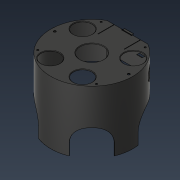
# Autodesk Inventor part: Gehäuse Mantel
Saved by Autodesk Inventor 2022.3 (Build 263350000, 350)
## iProperties
Part Number: Gehäuse Mantel
Material: Polyethylen, hohe Dichte
Document SubType Name: Modeling
Designer: rYan
Density: 0.952 g/cm^3
Appearance: Glatt - Schwarz
Mass: 76.0601 g
Surface Area: 1373.15 cm^2
Volume: 79.895 cm^3
Author: rYan
Autodesk Inventor part; units mm, degrees
ref_plane "XZ Plane" through (0, 0, 0) normal (0, 1, 0) x (-1, 0, 0)
ref_plane "XY Plane" through (0, 0, 0) normal (0, 0, 1) x (1, 0, 0)
sketch "Skizze1" plane through (0, 0, 0) normal (0, 0, 1) x (1, 0, 0)
  arc A0 (-44.0306, 77) -> (44.0306, 77) centre (0, 0) ccw
  circle A1 centre (0, 0) radius 25
  circle A2 centre (54.772, 35) radius 20
  circle A3 centre (-54.772, 35) radius 20
  circle A4 centre (-35, -54.772) radius 20
  circle A5 centre (35, -54.772) radius 20
  line L0 (0, 110.14) -> (0, -121.84) projected
  line L1 (-124.18, 0) -> (124.18, 0) projected
  line L2 (-44.0306, 77) -> (44.0306, 77)
  circle A6 centre (0, -59.5) radius 7.5
  circle A7 centre (0, 59.5) radius 7.5
  circle A8 centre (-80, 0) radius 2.2
  circle A9 centre (80, 0) radius 2.2
  dimension "d0" = 177.4
  dimension "d1" = 50
  dimension "d2" = 40
  dimension "d3" = 35
  dimension "d4" = 54.772
  dimension "d5" = 54.772
  dimension "d6" = 35
  dimension "d7" = 77
  dimension "d16" = 59.5
  dimension "d17" = 15
  dimension "d85" = 4.4
  dimension "d86" = 160
  constraints: 10 centre point, 4 point on line, 2 coincident, 2 end point, 2 equal radius, 2 point on circle, 1 horizontal, 4 other
  measures "d0" diameter of A0
  measures "d1" diameter of A1
  measures "d2" diameter of A2
  measures "d3" distance from line of A2.centre L1
  measures "d4" distance from line of A2.centre L0
  measures "d5" distance from line of L1 A5.centre
  measures "d6" distance from line of A5.centre L0
  measures "d7" distance between parallel lines of L2 L1
  measures "d16" distance from line of A6.centre L1
  measures "d17" diameter of A6
  measures "d85" diameter of A8
  measures "d86" distance of A9.centre A8.centre
extrude "Extrusion1" add sketch "Skizze1" along normal blind 1.2 contours L2 L0 A7 A1 L1 A8 A0 | L1 A8 A1 L0 A6 A0 | L2 A0 L1 A9 A1 L0 A7 | L0 A6 A1 L1 A9 A0 | A7 L0 | L0 A7 | A6 L0 | L0 A6
sketch "Skizze5" plane through (0, 0, 0) normal (0, 0, -1) x (-1, 0, 0)
  line L0 (-44.0306, 77) -> (44.0306, 77) projected
  line L1 (-29, 77) -> (29, 77)
  line L2 (29, 77) -> (29, -29)
  line L3 (-29, -29) -> (-29, 77)
  line L4 (0, -121.84) -> (0, 110.14) projected
  line L5 (-29, -29) -> (29, -29)
  circle A0 centre (0, 0) radius 25 projected
  circle A1 centre (-35, -54.772) radius 20 projected
  circle A2 centre (35, -54.772) radius 20 projected
  circle A3 centre (54.772, 35) radius 20 projected
  circle A4 centre (-54.772, 35) radius 20 projected
  arc A5 (-44.0306, 77) -> (44.0306, 77) centre (0, 0) ccw projected
  line L6 (-44.0306, 77) -> (44.0306, 77) projected
  circle A6 centre (-54.772, 35) radius 22
  circle A7 centre (54.772, 35) radius 22
  circle A8 centre (-35, -54.772) radius 22
  circle A9 centre (35, -54.772) radius 22
  line L7 (-44.0306, 77) -> (44.0306, 77) projected
  line L8 (30, -30) -> (-30, -30)
  line L9 (-30, -30) -> (-30, 77)
  line L10 (-30, 77) -> (30, 77)
  line L11 (30, 77) -> (30, -30)
  dimension "d18" = 58
  dimension "d19" = 29
  dimension "d43" = 44
  dimension "d45" = 44
  dimension "d46" = 44
  dimension "d47" = 44
  dimension "d221" = 106
  dimension "d228" = 1
  dimension "d229" = 1
  dimension "d230" = 1
  constraints: 16 end point, 4 centre point, 4 coincident, 3 horizontal, 3 parallel, 2 perpendicular, 2 point on line, 1 other
  measures "d18" distance between parallel lines of L2 L3
  measures "d19" distance from line of point (0, 0) L5
  measures "d43" diameter of A6
  measures "d45" diameter of A7
  measures "d46" diameter of A9
  measures "d47" diameter of A8
  measures "d221" distance of L3.start L1.start
  measures "d228" distance between parallel lines of L8 L5
  measures "d229" distance between parallel lines of L11 L2
  measures "d230" distance between parallel lines of L9 L3
extrude "Extrusion4" add sketch "Skizze5" along normal blind 1 contours L0 L3 L5 L4 L8 L9 | L4 L5 L2 L0 L11 L8
sketch "Skizze9" plane through (0, 0, -1) normal (0, 0, -1) x (-1, 0, 0)
  line L0 (-29, -29) -> (-29, 77) projected
  line L1 (29, -29) -> (-29, -29) projected
  line L2 (29, 77) -> (29, -29) projected
  line L3 (-29, 77) -> (-29, -29) projected
  line L4 (-29, 77) -> (-28, 77)
  line L5 (-28, 77) -> (-28, 42)
  line L6 (-28, 42) -> (-29, 42)
  line L7 (-29, 42) -> (-29, 77)
  line L8 (29, 77) -> (28, 77)
  line L9 (28, 77) -> (28, 42)
  line L10 (28, 42) -> (29, 42)
  line L11 (29, 42) -> (29, 77)
  line L12 (-29, 77) -> (29, 77) projected
  line L13 (29, 77) -> (29, -29) projected
  line L14 (-11, 75) -> (11, 75)
  line L15 (10, 76) -> (-10, 76)
  line L16 (-10, 76) -> (-10, 77)
  line L17 (-10, 77) -> (-11, 77)
  line L18 (-11, 77) -> (-11, 75)
  line L19 (-44.0306, 77) -> (44.0306, 77) projected
  line L20 (10, 76) -> (10, 77)
  line L21 (10, 77) -> (11, 77)
  line L22 (11, 77) -> (11, 75)
  line L23 (0, -121.84) -> (0, 110.14) projected
  point P0 (0, 0)
  dimension "d48" = 1
  dimension "d49" = 1
  dimension "d50" = 35
  dimension "d245" = 20
  dimension "d246" = 1
  dimension "d247" = 1
  dimension "d248" = 1
  constraints: 32 end point, 7 parallel, 5 collinear, 4 horizontal, 2 perpendicular, 2 point on line, 1 vertical, 4 other
  measures "d48" distance of L5.end L6.end
  measures "d49" distance of L9.end L10.end
  measures "d50" distance of L4.end L5.end
  measures "d245" distance of L15.start L15.end
  measures "d246" distance between parallel lines of L16 L18
  measures "d247" distance between parallel lines of L12 L15
  measures "d248" distance between parallel lines of L14 L15
extrude "Extrusion8" cut sketch "Skizze9" against normal through all contours L0 L4 L5 L6 | L23 L15 L20 L12 L22 L14 | L14 L18 L12 L16 L15 L23 | L10 L9 L8 L2
sketch "Skizze2" plane through (0, 0, 0) normal (0, 0, -1) x (-1, 0, 0)
  arc A0 (-44.0306, 77) -> (44.0306, 77) centre (0, 0) ccw projected
  line L0 (-44.0306, 77) -> (44.0306, 77) projected
  arc A1 (-43.7105, 75.8) -> (43.7105, 75.8) centre (0, 0) ccw
  line L1 (-43.7105, 75.8) -> (43.7105, 75.8)
  dimension "d10" = 1.2
  constraints: 2 end point, 2 point on circle, 1 centre point, 1 other
  measures "d10" radial gap between concentric circles of A0 A1
extrude "Extrusion2" add sketch "Skizze2" along normal blind 134.5
sketch "Skizze30" plane through (0, 0, 1.2) normal (0, 0, 1) x (1, 0, 0)
  line L0 (0, 117.34) -> (0, -123.04) projected
  line L1 (-124.18, 0) -> (124.18, 0) projected
  circle A0 centre (0, 0) radius 83 construction
  line L2 (0, 0) -> (-47.6068, 67.9896) construction
  line L3 (0, 0) -> (-63.5817, -53.3514) construction
  point P0 (63.5817, -53.3514)
  point P1 (47.6068, 67.9896)
  dimension "d144" = 166
  dimension "d145" = 40
  dimension "d146" = 55
  constraints: 4 end point, 4 point on circle, 3 coincident, 2 symmetric about line, 1 centre point
  measures "d144" diameter of A0
  measures "d145" angle of L1 L3
  measures "d146" angle of L2 L1
hole "Bohrung1" at (-47.6068, 67.9896, 1.2) at (-63.5817, -53.3514, 1.2) at (63.5817, -53.3514, 1.2) at (47.6068, 67.9896, 1.2) direction (0, 0, -1) diameter 3.3 end through all
ref_plane "Arbeitsebene7" through (0, 0, 0) normal (0.6427876, 0.7660444, 0) x (0, 0, 1)
sketch "Skizze34" plane through (0, 0, 0) normal (0.6427876, 0.7660444, 0) x (0, 0, 1)
  line L0 (-53.4, 0) -> (8.9, 0) projected
  line L1 (0, 33) -> (0, -5.5) projected
  line L2 (-26.8223, 2.5) -> (-37.1777, 2.5)
  line L3 (-37.1777, 2.5) -> (-44.5, 9.8223)
  line L4 (-44.5, 9.8223) -> (-44.5, 20.1777)
  line L5 (-44.5, 20.1777) -> (-37.1777, 27.5)
  line L6 (-37.1777, 27.5) -> (-26.8223, 27.5)
  line L7 (-26.8223, 27.5) -> (-19.5, 20.1777)
  line L8 (-19.5, 20.1777) -> (-19.5, 9.8223)
  line L9 (-19.5, 9.8223) -> (-26.8223, 2.5)
  point P0 (0, 0)
  point P1 (-32, 15)
  point P2 (-32, 15)
  dimension "d176" = 15
  dimension "d177" = 32
  dimension "d194" = 25
  constraints: 16 end point, 1 coincident, 1 horizontal, 17 other
  measures "d176" distance from line of point (-32, 15) L0
  measures "d177" distance from line of L1 point (-32, 15)
  measures "d194" distance between parallel lines of L2 L6
extrude "Extrusion24" cut sketch "Skizze34" along normal through all
sketch "Skizze40" plane through (29, 77, 1.2) normal (0, 1, 0) x (1, 0, 0)
  line L0 (0, 1.2) -> (0, 0) projected
  line L1 (15.0306, 0) -> (0, 0) projected
  line L2 (15.0306, 135.7) -> (15.0306, 0) projected
  line L3 (-73.0306, 135.7) -> (15.0306, 135.7) projected
  line L4 (-73.0306, 0) -> (-73.0306, 135.7) projected
  line L5 (-58, 0) -> (-73.0306, 0) projected
  line L6 (-58, 0) -> (-58, 1.2) projected
  line L7 (-57, 1.2) -> (-58, 1.2) projected
  line L8 (-57, 1.2) -> (-57, 0) projected
  line L9 (-1, 0) -> (-18, 0) projected
  line L10 (-1, 0) -> (-1, 1.2) projected
  line L11 (0, 1.2) -> (-1, 1.2) projected
  line L12 (-73.5306, 77.7) -> (-73.5306, 135.7)
  line L13 (-73.5306, 135.7) -> (15.5306, 135.7)
  line L14 (15.5306, 135.7) -> (15.5306, 77.7)
  line L15 (-29, 162.84) -> (-29, -27.14) projected
  line L16 (-69, 77.7) -> (-69, 57.7)
  line L17 (-69, 57.7) -> (11, 57.7)
  line L18 (11, 57.7) -> (11, 77.7)
  line L19 (15.5306, 77.7) -> (11, 77.7)
  line L20 (-69, 77.7) -> (-73.5306, 77.7)
  line L21 (-8, 31) -> (-2, 25)
  line L22 (-2, 25) -> (10, 25)
  line L23 (10, 25) -> (4, 31)
  line L24 (4, 31) -> (-8, 31)
  line L25 (-50, 31) -> (-56, 25)
  line L26 (-56, 25) -> (-68, 25)
  line L27 (-68, 25) -> (-62, 31)
  line L28 (-62, 31) -> (-50, 31)
  line L29 (-40, 0) -> (-57, 0) projected
  line L30 (-40, 0) -> (-40, 1.2) projected
  line L31 (-39, 1.2) -> (-40, 1.2) projected
  line L32 (-39, 1.2) -> (-39, 0) projected
  line L33 (-19, 0) -> (-39, 0) projected
  line L34 (-19, 0) -> (-19, 1.2) projected
  line L35 (-18, 1.2) -> (-19, 1.2) projected
  line L36 (-18, 1.2) -> (-18, 0) projected
  line L37 (-19, 1.2) -> (0, 1.2)
  line L38 (0, 1.2) -> (0, 4.2)
  line L39 (0, 4.2) -> (-19, 4.2)
  line L40 (-19, 4.2) -> (-19, 1.2)
  line L41 (-58, 1.2) -> (-39, 1.2)
  line L42 (-39, 1.2) -> (-39, 4.2)
  line L43 (-39, 4.2) -> (-58, 4.2)
  line L44 (-58, 4.2) -> (-58, 1.2)
  line L45 (1, 28) -> (-59, 28) construction
  dimension "d236" = 0.5
  dimension "d237" = 58
  dimension "d238" = 20
  dimension "d239" = 80
  dimension "d240" = 45
  dimension "d241" = 25
  dimension "d243" = 6
  dimension "d244" = 12
  dimension "d249" = 3
  dimension "d252" = 60
  dimension "d253" = 3
  dimension "d254" = 3
  constraints: 50 end point, 10 parallel, 8 horizontal, 5 collinear, 4 perpendicular, 8 other
  measures "d236" distance between parallel lines of L12 L4
  measures "d237" distance of L12.start L12.end
  measures "d238" distance of L16.start L16.end
  measures "d239" distance of L16.end L17.end
  measures "d240" angle of L23 L24
  measures "d241" distance between parallel lines of L9 L22
  measures "d243" distance between parallel lines of L22 L24
  measures "d244" distance of L23.end L21.start
  measures "d249" distance of L39.end L34.end
  measures "d252" distance of L45.start L45.end
  measures "d253" horizontal distance of L45.start L21.end
  measures "d254" horizontal distance of L45.end L25.end
extrude "Extrusion28" cut sketch "Skizze40" against normal blind 2 contours L11 L37 L35 L40 L39 L38 | L19 L18 L17 L15 L3 L2 | L2 L13 L14 L19 | L15 L17 L16 L20 L4 L3 | L4 L20 L12 L13 | L31 L41 L7 L44 L43 L42 | L24 L23 L22 L21 | L25 L26 L27 L28
chamfer "Fase13" distance 1 angle 45 5 edges at (-74.772, 35, 1.2) (-25, 0, 1.2) (15, -54.772, 1.2) (34.772, 35, 1.2) (-55, -54.772, 1.2)
chamfer "Fase14" distance 0.3 angle 45 6 edges at (77.8, 0, 1.2) (63.5817, -51.7014, 1.2) (47.6068, 69.6396, 1.2) (-47.6068, 69.6396, 1.2) (-82.2, 0, 1.2) (-63.5817, -51.7014, 1.2)
sketch "Skizze39" plane through (0, 0, 0) normal (0, 0, -1) x (-1, 0, 0)
  line L0 (-30, 75.8) -> (-43.7105, 75.8) projected
  line L1 (-28, 77) -> (-28, 42) projected
  line L2 (-28, 42) -> (-29, 42) projected
  line L3 (-29, 42) -> (-29, -29) projected
  line L4 (-29, -29) -> (29, -29) projected
  line L5 (29, -29) -> (29, 42) projected
  line L6 (29, 42) -> (28, 42) projected
  line L7 (28, 42) -> (28, 77) projected
  circle A0 centre (0, 0) radius 25 projected
  arc A1 (-43.7105, 75.8) -> (43.7105, 75.8) centre (0, 0) ccw projected
  line L8 (43.7105, 75.8) -> (30, 75.8) projected
  line L9 (30, 75.8) -> (30, -30) projected
  line L10 (30, -30) -> (-30, -30) projected
  line L11 (-30, -30) -> (-30, 75.8) projected
  line L12 (11, 77) -> (28, 77) projected
  line L13 (11, 77) -> (11, 75) projected
  line L14 (11, 75) -> (-11, 75) projected
  line L15 (-11, 75) -> (-11, 77) projected
  line L16 (-28, 77) -> (-11, 77) projected
extrude "Extrusion27" cut sketch "Skizze39" against normal blind 0.2 contours L16 L15 L14 L13 L12 L7 L6 L5 L4 L3 L2 L1
chamfer "Fase15" distance 2 angle 45 4 edges at (29, 76.4, -3) (10, 76.4, -3) (-10, 76.4, -3) (-29, 76.4, -3)
fillet "Rundung3" radius 4 4 edges at (40, 76.4, -56.5) (40, 76.4, -76.5) (-40, 76.4, -56.5) (-40, 76.4, -76.5)
sketch "Skizze41" plane through (-44.0306, 77, 1.2) normal (0, 1, 0) x (1, 0, 0)
  line L0 (54.0306, 0) -> (34.0306, 0) projected
  line L1 (54.0306, 0) -> (54.0306, 2.2) projected
  line L2 (34.0306, 2.2) -> (34.0306, 0) projected
  line L3 (54.0306, 0) -> (34.0306, 0)
  line L4 (34.0306, 0) -> (34.0306, 0.2)
  line L5 (34.0306, 0.2) -> (54.0306, 0.2)
  line L6 (54.0306, 0.2) -> (54.0306, 0)
  point P0 (44.0306, 1.2)
  dimension "d259" = 0.2
  constraints: 8 end point, 2 parallel, 1 horizontal, 1 perpendicular, 1 point on line
  measures "d259" distance between parallel lines of L0 L5
extrude "Extrusion29" add sketch "Skizze41" along normal blind 4
sketch "Skizze42" plane through (0, 0, -134.5) normal (0, 0, -1) x (-1, 0, 0)
  line L0 (-44.5306, 75.3212) -> (-44.5306, 76.7119) projected
  arc A0 (-44.5306, 76.7119) -> (44.5306, 76.7119) centre (0, 0) ccw projected
  line L1 (44.5306, 76.7119) -> (44.5306, 75.3212) projected
  arc A1 (-44.5306, 75.3212) -> (44.5306, 75.3212) centre (0, 0) ccw projected
  line L2 (0, 0) -> (-76.0307, 45.6839) construction
  arc A2 (-70.9774, 53.1967) -> (-75.2721, 46.9234) centre (0, 0) ccw construction
  line L3 (0, 0) -> (-62.7204, -62.7204) construction
  arc A3 (-44.5306, 76.7119) -> (44.5306, 76.7119) centre (0, 0) ccw construction
  line L4 (-124.18, 0) -> (124.18, 0) construction
  line L5 (0, 0) -> (-87.8368, 12.3447) construction
  line L6 (0, 0) -> (-82.2412, -33.2276) construction
  line L7 (0, 0) -> (-33.2276, -82.2412) construction
  arc A4 (-43.7105, 75.8) -> (43.7105, 75.8) centre (0, 0) ccw projected
  line L8 (-86.6485, 12.1776) -> (-87.8368, 12.3447)
  line L9 (-81.1286, -32.7781) -> (-82.2412, -33.2276)
  line L10 (-32.7781, -81.1286) -> (-33.2276, -82.2412)
  arc A5 (-44.5306, 76.7119) -> (-87.8368, 12.3447) centre (0, 0) ccw
  arc A6 (-44.5306, 75.3212) -> (-86.6485, 12.1776) centre (0, 0) ccw
  line L11 (-44.5306, 75.3212) -> (-44.5306, 76.7119) projected
  line L12 (-44.5306, 76.7119) -> (-44.5306, 75.3212)
  arc A7 (-82.2412, -33.2276) -> (-33.2276, -82.2412) centre (0, 0) ccw
  arc A8 (-81.1286, -32.7781) -> (-32.7781, -81.1286) centre (0, 0) ccw
  dimension "d262" = 31
  dimension "d263" = 45
  dimension "d264" = 23
  dimension "d265" = 23
  constraints: 18 end point, 14 point on circle, 4 centre point, 4 collinear, 4 point on line, 2 coincident, 1 midpoint, 6 other
  measures "d262" angle of L2 L4
  measures "d263" angle of L3 L4
  measures "d264" angle of L6 L3
  measures "d265" angle of L5 L2
extrude "Extrusion30" cut sketch "Skizze42" against normal blind 58 contours A1 L8 A0 L0 | A1 L10 A0 L9
mirror "Spiegeln2" about plane through (0, 0, 0) normal (1, 0, 0) of "Extrusion30"
fillet "Rundung4" radius 34 6 edges at (87.2426, 12.2612, -76.5) (81.6849, -33.0028, -76.5) (33.0028, -81.6849, -76.5) (-33.0028, -81.6849, -76.5) (-81.6849, -33.0028, -76.5) (-87.2426, 12.2612, -76.5)
equation "\"d5\" = d4"
equation "\"d6\" = d3"
equation "\"d19\" = 0.5 * d18"
equation "\"d45\" = d43"
equation "\"d46\" = d43"
equation "\"d47\" = d43"
